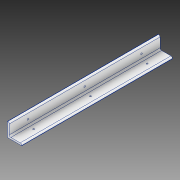
# Autodesk Inventor part: 4104b_Aluminum Box DividerAngle_V1
Saved by Autodesk Inventor 2020 (Build 240168000, 168)
## iProperties
Created: 2020-09-13
Part Number: 4104b_Aluminum Box DividerAngle_V1
Material: Aluminum 6061
Document SubType Name: Modeling
Designer: Eli Mattingly
Density: 2.7 g/cm^3
Appearance: Aluminum - Flat
Author: Eli Mattingly
Autodesk Inventor part; units mm, degrees
ref_plane "YZ Plane" through (0, 0, 0) normal (1, 0, 0) x (0, 1, 0)
ref_plane "XZ Plane" through (0, 0, 0) normal (0, 1, 0) x (-1, 0, 0)
ref_plane "XY Plane" through (0, 0, 0) normal (0, 0, 1) x (1, 0, 0)
sketch "Sketch1" plane through (0, 0, 0) normal (0, 0, 1) x (1, 0, 0)
  line L0 (-19.05, -19.05) -> (19.05, -19.05)
  line L1 (19.05, -19.05) -> (19.05, 19.05)
  line L2 (19.05, 19.05) -> (-19.05, 19.05)
  line L3 (-19.05, 19.05) -> (-19.05, -19.05)
  line L4 (-19.05, -19.05) -> (19.05, 19.05) construction
  line L5 (19.05, -19.05) -> (-19.05, 19.05) construction
  line L6 (19.05, 19.05) -> (-14.2748, 19.05)
  line L7 (-14.2748, 19.05) -> (-14.2748, -14.2748)
  line L8 (-14.2748, -14.2748) -> (19.05, -14.2748)
  line L9 (19.05, -14.2748) -> (19.05, 19.05)
  point P0 (0, 0)
  point P1 (-14.2748, 19.05)
  dimension "d0" = 38.1
  dimension "d1" = 38.1
  dimension "d2" = 4.7752
  dimension "d3" = 4.7752
  constraints: 20 end point, 4 parallel, 2 horizontal, 2 midpoint, 2 perpendicular
  measures "d0" distance of L2.end L1.end
  measures "d1" distance of L1.end L0.end
  measures "d2" distance between parallel lines of L3 L7
  measures "d3" distance between parallel lines of L0 L8
extrude "Extrusion1" add sketch "Sketch1" along normal mid plane 405 contours L3 L2 L7 L8 L1 L0
sketch "Sketch2" plane through (-14.2748, -14.2748, 202.5) normal (1, 0, 0) x (0, 0, -1)
  line L0 (0, 0) -> (0, 33.3248) projected
  line L1 (405, 33.3248) -> (405, 0) projected
  line L2 (0, 15.2248) -> (405, 15.2248)
  line L3 (405, -4.7752) -> (0, -4.7752) projected
  point P0 (202.5, 14.2748)
  point P1 (202.5, 15.2248)
  point P2 (50, 15.2248)
  point P3 (355, 15.2248)
  dimension "d6" = 20
  dimension "d7" = 50
  dimension "d8" = 50
  constraints: 4 point on line, 2 end point, 1 horizontal, 1 midpoint
  measures "d6" distance between parallel lines of L3 L2
  measures "d7" distance from line of L0 point (50, 15.225)
  measures "d8" distance from line of L1 point (355, 15.225)
hole "Hole1" at (-14.2748, 0.95, 0) at (-14.2748, 0.95, 152.5) at (-14.2748, 0.95, -152.5) direction (-1, 0, 0) diameter 4 end through all
ref_plane "Work Plane1" through (-14.2748, -14.2748, 202.5) normal (-0.7071068, 0.7071068, 0) x (0, 0, 1)
mirror "Mirror1" about plane through (-14.2748, -14.2748, 202.5) normal (-0.7071068, 0.7071068, 0) of "Hole1"
fillet "Fillet1" radius 4 3 edges at (-14.2748, 19.05, 0) (-14.2748, -14.2748, 0) (19.05, -14.2748, 0)
equation "\"d3\" = d2"
equation "\"d8\" = d7"
body "Solid1"
